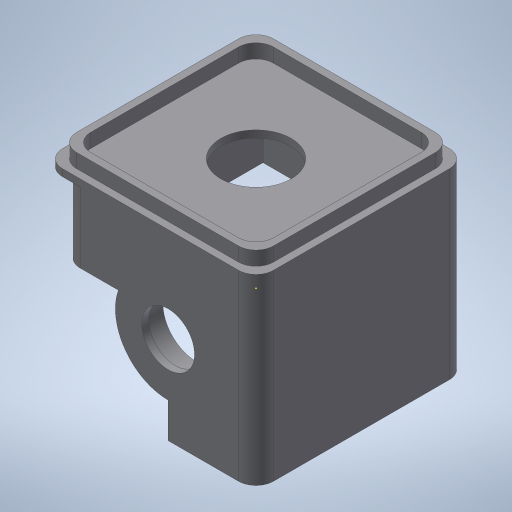
# Autodesk Inventor part: Pieza 2.3 final
Saved by Autodesk Inventor 2023.1 (Build 271208000, 208)
## iProperties
Created: 2022-10-20
Part Number: Pieza 2.3 final
Material: Generic
Document SubType Name: Modeling
Designer: User
Density: 1 g/cm^3
Appearance: Default
Author: User
Autodesk Inventor part; units mm, degrees
ref_plane "YZ Plane" through (0, 0, 0) normal (1, 0, 0) x (0, 1, 0)
ref_plane "XZ Plane" through (0, 0, 0) normal (0, 1, 0) x (-1, 0, 0)
ref_plane "XY Plane" through (0, 0, 0) normal (0, 0, 1) x (1, 0, 0)
sketch "Sketch1" plane through (0, 0, 0) normal (0, 1, 0) x (-1, 0, 0)
  line L0 (0, 0) -> (60, 0)
  line L1 (60, 0) -> (60, 60)
  line L2 (60, 60) -> (0, 60)
  line L3 (0, 60) -> (0, 0)
  dimension "d0" = 60
  dimension "d1" = 60
  constraints: 8 end point, 2 parallel, 1 horizontal, 1 perpendicular
  measures "d0" distance of L2.end L1.end
  measures "d1" distance of L1.end L0.end
extrude "Extrusion1" add sketch "Sketch1" along normal blind 2
sketch "Sketch2" plane through (0, 2, 0) normal (0, 1, 0) x (1, 0, 0)
  line L0 (-60, 0) -> (-60, -60) projected
  line L1 (-60, -60) -> (0, -60) projected
  line L2 (0, -60) -> (0, 0) projected
  line L3 (0, 0) -> (-60, 0) projected
  line L4 (-58, -2) -> (-58, -58)
  line L5 (-58, -58) -> (-2, -58)
  line L6 (-2, -58) -> (-2, -2)
  line L7 (-2, -2) -> (-58, -2)
  line L8 (-56, -4) -> (-56, -56)
  line L9 (-56, -56) -> (-4, -56)
  line L10 (-4, -56) -> (-4, -4)
  line L11 (-4, -4) -> (-56, -4)
  dimension "d4" = 2
  dimension "d5" = 2
  constraints: 16 end point, 6 other
  measures "d4" distance between parallel lines of L3 L7
  measures "d5" distance between parallel lines of L7 L11
extrude "Extrusion2" add sketch "Sketch2" along normal blind 4 contours L7 L6 L5 L4
sketch "Sketch3" plane through (0, 2, 0) normal (0, 1, 0) x (1, 0, 0)
  line L0 (0, 0) -> (-60, 0) construction
  line L1 (-60, 0) -> (-60, -60) construction
  line L2 (0, 0) -> (-60, -60) construction
  line L3 (-60, -60) -> (0, -60) construction
  line L4 (0, -60) -> (-60, 0) construction
  circle A0 centre (-30, -30) radius 10
  dimension "d8" = 20
  constraints: 4 end point, 1 centre point, 1 coincident, 1 midpoint
  measures "d8" diameter of A0
hole "Hole1" at (-30, 2, 30) direction (0, -1, 0) diameter 20 depth 8 tip angle 118
sketch "Sketch4" plane through (0, 0, 0) normal (0, -1, 0) x (1, 0, 0)
  circle A0 centre (-30, 30) radius 10 projected
  line L0 (-60, 0) -> (-60, 60) projected
  line L1 (0, 0) -> (-60, 0) projected
  line L2 (0, 60) -> (0, 0) projected
  line L3 (-60, 60) -> (0, 60) projected
  line L4 (0, 0) -> (-50, 0)
  line L5 (-50, 0) -> (-50, 8)
  line L6 (-50, 8) -> (0, 8)
  line L7 (0, 8) -> (0, 0)
  line L8 (0, 60) -> (-50, 60)
  line L9 (-50, 60) -> (-50, 52)
  line L10 (-50, 52) -> (0, 52)
  line L11 (0, 52) -> (0, 60)
  line L12 (0, 8) -> (-5, 8)
  line L13 (-5, 8) -> (-5, 52)
  line L14 (-5, 52) -> (0, 52)
  line L15 (0, 52) -> (0, 8)
  dimension "d16" = 50
  dimension "d17" = 8
  dimension "d18" = 50
  dimension "d19" = 8
  dimension "d20" = 5
  constraints: 24 end point, 6 parallel, 3 horizontal, 3 perpendicular, 1 point on line
  measures "d16" distance of L5.end L6.end
  measures "d17" distance of L4.end L5.end
  measures "d18" distance of L10.end L9.end
  measures "d19" distance of L9.end L8.end
  measures "d20" distance of L13.end L14.end
extrude "Extrusion3" add sketch "Sketch4" along normal blind 10 contours L5 L6 L2 L1 | L3 L2 L10 L9 | L6 L13 L10 L2
sketch "Sketch5" plane through (-5, 0, 52) normal (0, 0, -1) x (-1, 0, 0)
  line L0 (55, 0) -> (45, 0) projected
  line L1 (45, 0) -> (45, -10) projected
  line L2 (-5, -10) -> (45, -10) projected
  line L3 (-5, -10) -> (-5, 2) projected
  line L4 (55, 2) -> (-5, 2) projected
  line L5 (55, 0) -> (55, 2) projected
  line L6 (-5, -10) -> (45, -10) construction
  line L7 (-5, -10) -> (5, -10) construction
  line L8 (5, -10) -> (20, -10) construction
  line L9 (20, -10) -> (20, -25) construction
  circle A0 centre (20, -25) radius 15
  point P0 (-5, 0)
  dimension "d23" = 10
  dimension "d24" = 15
  dimension "d25" = 15
  dimension "d26" = 30
  constraints: 6 end point, 1 centre point, 1 coincident, 1 midpoint, 1 perpendicular, 1 point on line
  measures "d23" distance of L2.start L7.end
  measures "d24" distance of L7.end L8.end
  measures "d25" distance of L8.end L9.end
  measures "d26" diameter of A0
extrude "Extrusion4" add sketch "Sketch5" against normal blind 8 contours A0
sketch "Sketch6" plane through (-50, 0, 8) normal (0, 0, 1) x (1, 0, 0)
  line L0 (0, 0) -> (-10, 0) projected
  line L1 (-10, 0) -> (-10, 2) projected
  line L2 (50, 2) -> (-10, 2) projected
  line L3 (50, -10) -> (50, 2) projected
  line L4 (0, -10) -> (50, -10) projected
  line L5 (0, 0) -> (0, -10) projected
  line L6 (0, -10) -> (50, -10) construction
  line L7 (50, -10) -> (40, -10) construction
  line L8 (40, -10) -> (25, -10) construction
  line L9 (25, -10) -> (25, -25) construction
  circle A0 centre (25, -25) radius 15
  point P0 (50, 0)
  dimension "d29" = 10
  dimension "d30" = 15
  dimension "d31" = 15
  dimension "d32" = 30
  constraints: 6 end point, 1 centre point, 1 coincident, 1 midpoint, 1 perpendicular, 1 point on line
  measures "d29" distance of L3.start L7.end
  measures "d30" distance of L7.end L8.end
  measures "d31" distance of L8.end L9.end
  measures "d32" diameter of A0
extrude "Extrusion5" add sketch "Sketch6" against normal blind 8 contours A0
sketch "Sketch7" plane through (-25, -25, 52) normal (0, 0, -1) x (-1, 0, 0)
  circle A0 centre (0, 0) radius 15 projected
  circle A1 centre (0, 0) radius 13.5
  circle A2 centre (0, 0) radius 11.5
  circle A3 centre (0, 0) radius 15
  circle A4 centre (0, 0) radius 15 projected
  line L0 (0, -15) -> (0, 15)
  line L1 (15, 0) -> (-15, 0)
  line L2 (0, 0) -> (-12.9904, -7.5)
  line L3 (0, 0) -> (15, 0) construction
  line L4 (-12.9904, -7.5) -> (12.9904, 7.5)
  line L5 (0, 0) -> (-7.5, -12.9904)
  line L6 (0, 0) -> (15, 0) construction
  line L7 (-7.5, -12.9904) -> (7.5, 12.9904)
  line L8 (0, 0) -> (7.5, -12.9904)
  line L9 (0, 0) -> (15, 0) construction
  line L10 (7.5, -12.9904) -> (-7.5, 12.9904)
  line L11 (0, 0) -> (12.9904, -7.5)
  line L12 (0, 0) -> (15, 0) construction
  line L13 (12.9904, -7.5) -> (-12.9904, 7.5)
  point P0 (-25, 25)
  point P1 (11.6913, 6.75)
  point P2 (9.9593, 5.75)
  point P3 (11.5, 0)
  point P4 (13.5, 0)
  point P5 (5.75, 9.9593)
  point P6 (6.75, 11.6913)
  point P7 (0, 13.5)
  point P8 (0, 11.5)
  point P9 (-11.6913, 6.75)
  point P10 (-9.9593, 5.75)
  point P11 (-5.75, 9.9593)
  point P12 (-6.75, 11.6913)
  point P13 (-11.6913, -6.75)
  point P14 (-9.9593, -5.75)
  point P15 (-11.5, 0)
  point P16 (-13.5, 0)
  point P17 (-5.75, -9.9593)
  point P18 (-6.75, -11.6913)
  point P19 (0, -13.5)
  point P20 (0, -11.5)
  point P21 (11.6913, -6.75)
  point P22 (9.9593, -5.75)
  point P23 (5.75, -9.9593)
  point P24 (6.75, -11.6913)
  dimension "d35" = 1.5
  dimension "d36" = 2
  dimension "d37" = 30
  dimension "d38" = 150
  dimension "d39" = 120
  dimension "d40" = 60
  dimension "d41" = 30
  constraints: 28 end point, 5 horizontal, 4 equal length, 3 centre point, 3 point on line, 1 coincident, 1 vertical, 1 vertical alignment, 12 other
  measures "d36" radial gap between concentric circles of A1 A2
  measures "d37" diameter of A3
  measures "d38" angle of L2 L3
  measures "d39" angle of L5 L6
  measures "d40" angle of L8 L9
  measures "d41" angle of L11 L12
extrude "Extrusion6" cut sketch "Sketch7" against normal blind 5 contours L1 A2 L4 A1 | A1 L8 A2 L11 | L7 A2 L0 A1 | A1 L5 A2 L0 | A2 L2 A1 L1 | A2 L13 A1 L10
sketch "Sketch8" plane through (-25, -25, 8) normal (0, 0, 1) x (1, 0, 0)
  circle A0 centre (0, 0) radius 15
  circle A1 centre (0, 0) radius 13.5
  circle A2 centre (0, 0) radius 11.5
  circle A3 centre (0, 0) radius 15
  circle A4 centre (0, 0) radius 15
  line L0 (0, -15) -> (0, 15)
  line L1 (15, 0) -> (-15, 0)
  line L2 (0, 0) -> (-12.9904, -7.5)
  line L3 (0, 0) -> (15, 0) construction
  line L4 (-12.9904, -7.5) -> (12.9904, 7.5)
  line L5 (0, 0) -> (-7.5, -12.9904)
  line L6 (0, 0) -> (15, 0) construction
  line L7 (-7.5, -12.9904) -> (7.5, 12.9904)
  line L8 (0, 0) -> (7.5, -12.9904)
  line L9 (0, 0) -> (15, 0) construction
  line L10 (7.5, -12.9904) -> (-7.5, 12.9904)
  line L11 (0, 0) -> (12.9904, -7.5)
  line L12 (0, 0) -> (15, 0) construction
  line L13 (12.9904, -7.5) -> (-12.9904, 7.5)
  point P0 (25, 25)
  point P1 (-25, 25)
  point P2 (11.6913, 6.75)
  point P3 (9.9593, 5.75)
  point P4 (11.5, 0)
  point P5 (13.5, 0)
  point P6 (5.75, 9.9593)
  point P7 (6.75, 11.6913)
  point P8 (0, 13.5)
  point P9 (0, 11.5)
  point P10 (-11.6913, 6.75)
  point P11 (-9.9593, 5.75)
  point P12 (-5.75, 9.9593)
  point P13 (-6.75, 11.6913)
  point P14 (-11.6913, -6.75)
  point P15 (-9.9593, -5.75)
  point P16 (-11.5, 0)
  point P17 (-13.5, 0)
  point P18 (-5.75, -9.9593)
  point P19 (-6.75, -11.6913)
  point P20 (0, -13.5)
  point P21 (0, -11.5)
  point P22 (11.6913, -6.75)
  point P23 (9.9593, -5.75)
  point P24 (5.75, -9.9593)
  point P25 (6.75, -11.6913)
  point P26 (9.9593, -5.75)
  point P27 (11.6913, -6.75)
  point P28 (13.5, 0)
  point P29 (11.5, 0)
  point P30 (6.75, 11.6913)
  point P31 (5.75, 9.9593)
  point P32 (9.9593, 5.75)
  point P33 (11.6913, 6.75)
  point P34 (-6.75, 11.6913)
  point P35 (-5.75, 9.9593)
  point P36 (0, 11.5)
  point P37 (0, 13.5)
  point P38 (-9.9593, 5.75)
  point P39 (-11.6913, 6.75)
  point P40 (-13.5, 0)
  point P41 (-11.5, 0)
  point P42 (-6.75, -11.6913)
  point P43 (-5.75, -9.9593)
  point P44 (-9.9593, -5.75)
  point P45 (-11.6913, -6.75)
  point P46 (6.75, -11.6913)
  point P47 (5.75, -9.9593)
  point P48 (0, -11.5)
  point P49 (0, -13.5)
  dimension "d44" = 1.5
  dimension "d45" = 2
  dimension "d46" = 30
  dimension "d47" = 150
  dimension "d48" = 120
  dimension "d49" = 60
  dimension "d50" = 30
  constraints: 28 end point, 5 horizontal, 4 equal length, 3 centre point, 3 point on line, 1 coincident, 1 vertical, 1 vertical alignment, 14 other
  measures "d45" radial gap between concentric circles of A1 A2
  measures "d46" diameter of A3
  measures "d47" angle of L2 L3
  measures "d48" angle of L5 L6
  measures "d49" angle of L8 L9
  measures "d50" angle of L11 L12
extrude "Extrusion7" cut sketch "Sketch8" against normal blind 5 contours A1 L11 A2 L1 | L4 A2 L7 A1 | A1 L0 A2 L8 | L0 A2 L10 A1 | L1 A1 L13 A2 | A2 L5 A1 L2
sketch "Sketch9" plane through (-25, -25, 52) normal (0, 0, -1) x (-1, 0, 0)
  circle A0 centre (0, 0) radius 15 projected
  circle A1 centre (0, 0) radius 7.5
  point P0 (-25, 25)
  point P1 (0, 15)
  dimension "d53" = 15
  constraints: 1 centre point, 1 coincident, 1 vertical alignment
  measures "d53" diameter of A1
hole "Hole2" at (-25, -25, 52) direction (0, 0, 1) diameter 15 depth 8 tip angle 118
sketch "Sketch10" plane through (-25, -25, 8) normal (0, 0, 1) x (1, 0, 0)
  circle A0 centre (0, 0) radius 15 projected
  point P0 (25, 25)
  point P1 (0, 15)
  constraints: 1 coincident, 1 vertical alignment
hole "Hole3" at (-25, -25, 8) direction (0, 0, -1) diameter 15 depth 8 tip angle 118
sketch "Sketch11" plane through (-25, -25, 8) normal (0, 0, 1) x (1, 0, 0)
  circle A0 centre (0, 0) radius 7.5 projected
  circle A1 centre (0, 0) radius 15 projected
  circle A2 centre (0, 0) radius 9.5
  point P0 (25, 25)
  point P1 (0, 15)
  dimension "d68" = 2
  constraints: 1 centre point, 1 vertical alignment
  measures "d68" radial gap between concentric circles of A0 A2
extrude "Extrusion8" cut sketch "Sketch11" against normal blind 6 contours A2
sketch "Sketch12" plane through (-25, -25, 52) normal (0, 0, -1) x (-1, 0, 0)
  circle A0 centre (0, 0) radius 7.5 projected
  circle A1 centre (0, 0) radius 15 projected
  circle A2 centre (0, 0) radius 9.5
  point P0 (-25, 25)
  point P1 (0, 15)
  dimension "d71" = 2
  constraints: 1 centre point, 1 vertical alignment
  measures "d71" radial gap between concentric circles of A0 A2
extrude "Extrusion9" cut sketch "Sketch12" against normal blind 6 contours A2
sketch "Sketch13" plane through (-60, 2, 60) normal (0, 0, 1) x (1, 0, 0)
  point P0 (60, -2)
sketch "Sketch14" plane through (-60, 2, 60) normal (0, 0, 1) x (1, 0, 0)
  line L0 (0, -2) -> (10, -2) projected
  line L1 (10, -2) -> (10, -12) projected
  line L2 (35, -12) -> (10, -12) projected
  line L3 (60, -12) -> (35, -12) projected
  line L4 (60, -12) -> (60, 0) projected
  line L5 (0, 0) -> (60, 0) projected
  line L6 (0, -2) -> (0, 0) projected
  arc A0 (44.9593, -21.25) -> (40.75, -17.0407) centre (35, -27) ccw projected
  circle A1 centre (35, -27) radius 15 projected
  line L7 (60, -12) -> (60, 0) projected
  line L8 (60, -12) -> (35, -12)
  line L9 (35, -42) -> (35, -52)
  line L10 (35, -52) -> (60, -52)
  line L11 (60, -52) -> (60, -12)
  arc A2 (35, -42) -> (35, -12) centre (35, -27) ccw
  point P0 (60, -2)
  dimension "d74" = 25
  dimension "d75" = 40
  constraints: 8 end point, 2 parallel, 2 point on circle, 1 centre point, 1 coincident, 1 horizontal, 1 perpendicular, 1 other
  measures "d74" distance of L10.end L9.end
  measures "d75" distance of L9.end L8.end
extrude "Extrusion10" add sketch "Sketch14" against normal blind 8 contours L3 L11 L10 L9 A1
sketch "Sketch15" plane through (0, 2, 0) normal (0, 0, -1) x (-1, 0, 0)
  line L0 (50, -2) -> (60, -2) projected
  line L1 (60, -2) -> (60, 0) projected
  line L2 (0, 0) -> (60, 0) projected
  line L3 (0, -12) -> (0, 0) projected
  line L4 (25, -12) -> (0, -12) projected
  line L5 (50, -12) -> (25, -12) projected
  line L6 (50, -2) -> (50, -12) projected
  circle A0 centre (25, -27) radius 15 projected
  line L7 (0, -52) -> (25, -52) projected
  line L8 (25, -12) -> (0, -12)
  line L9 (0, -12) -> (0, -52)
  line L10 (0, -52) -> (25, -52)
  circle A1 centre (25, -27) radius 7.5 projected
  arc A2 (25, -12) -> (25, -42) centre (25, -27) ccw
  line L11 (25, -52) -> (25, -42)
  point P0 (0, -2)
  constraints: 8 end point, 2 parallel, 2 point on circle, 1 centre point, 1 coincident, 1 horizontal, 1 perpendicular, 2 other
extrude "Extrusion11" add sketch "Sketch15" against normal blind 8 contours A0 L11 L7 L9 L4
sketch "Sketch16" plane through (0, -10, 0) normal (0, -1, 0) x (1, 0, 0)
  line L0 (-4, 56) -> (-4, 4) projected
  line L1 (0, 8) -> (0, 52) projected
  line L2 (-5, 52) -> (-5, 8) projected
  line L3 (-25, 8) -> (0, 8) projected
  line L4 (0, 52) -> (-25, 52) projected
  line L5 (-5, 8) -> (-5, 52) projected
  line L6 (0, 8) -> (-5, 8)
  line L7 (-5, 8) -> (-5, 52)
  line L8 (-5, 52) -> (0, 52)
  line L9 (0, 52) -> (0, 8)
  point P0 (0, 0)
  constraints: 8 end point, 2 parallel, 1 horizontal, 1 perpendicular
extrude "Extrusion12" add sketch "Sketch16" along normal blind 40
sketch "Sketch17" plane through (0, 0, 0) normal (0, -1, 0) x (1, 0, 0)
  line L0 (-50, 52) -> (-50, 60) projected
  line L1 (-60, 60) -> (-50, 60) projected
  line L2 (-60, 0) -> (-60, 60) projected
  line L3 (-50, 0) -> (-60, 0) projected
  line L4 (-50, 0) -> (-50, 8) projected
  line L5 (-50, 8) -> (-5, 8) projected
  line L6 (-5, 8) -> (-5, 52) projected
  line L7 (-5, 52) -> (-50, 52) projected
  circle A0 centre (-30, 30) radius 10 projected
  line L8 (-50, 60) -> (-50, 52) projected
  line L9 (-50, 60) -> (-55, 60)
  line L10 (-55, 60) -> (-55, 0)
  line L11 (-55, 0) -> (-50, 0)
  line L12 (-50, 0) -> (-50, 60)
  point P0 (0, 0)
  dimension "d82" = 5
  dimension "d83" = 60
  constraints: 8 end point, 2 parallel, 1 horizontal, 1 perpendicular
  measures "d82" distance of L11.end L10.end
  measures "d83" distance of L10.end L9.end
extrude "Extrusion13" add sketch "Sketch17" along normal blind 20 contours L12 L4 L3 L10 L1 L0
sketch "Sketch18" plane through (0, 2, 0) normal (0, 0, -1) x (-1, 0, 0)
  circle A0 centre (25, -27) radius 7.5 projected
  line L0 (55, -2) -> (60, -2) projected
  line L1 (60, -2) -> (60, 0) projected
  line L2 (0, 0) -> (60, 0) projected
  line L3 (0, -52) -> (0, 0) projected
  line L4 (0, -52) -> (25, -52) projected
  line L5 (25, -52) -> (25, -42) projected
  arc A1 (25, -42) -> (25, -12) centre (25, -27) ccw projected
  line L6 (50, -12) -> (25, -12) projected
  line L7 (50, -12) -> (50, -22) projected
  line L8 (55, -22) -> (50, -22) projected
  line L9 (55, -2) -> (55, -22) projected
  line L10 (50, -12) -> (50, -22) projected
  line L11 (50, -12) -> (25, -12)
  line L12 (50, -22) -> (50, -12)
  arc A2 (39.1421, -22) -> (25, -12) centre (25, -27) ccw
  line L13 (39.1421, -22) -> (50, -22)
  point P0 (0, -2)
  constraints: 7 end point, 2 point on circle, 1 centre point, 1 coincident, 1 horizontal, 1 parallel
extrude "Extrusion14" add sketch "Sketch18" against normal blind 8 contours L13 A1 L6 L7
sketch "Sketch19" plane through (-60, 2, 60) normal (0, 0, 1) x (1, 0, 0)
  circle A0 centre (35, -27) radius 7.5 projected
  arc A1 (35, -12) -> (35, -42) centre (35, -27) ccw projected
  line L0 (35, -42) -> (35, -52) projected
  line L1 (35, -52) -> (60, -52) projected
  line L2 (60, -52) -> (60, 0) projected
  line L3 (0, 0) -> (60, 0) projected
  line L4 (0, -2) -> (0, 0) projected
  line L5 (0, -2) -> (5, -2) projected
  line L6 (5, -2) -> (5, -22) projected
  line L7 (10, -22) -> (5, -22) projected
  line L8 (10, -12) -> (10, -22) projected
  line L9 (35, -12) -> (10, -12) projected
  line L10 (35, -22) -> (35, -19.5)
  line L11 (35, -12) -> (10, -12)
  line L12 (10, -12) -> (10, -22)
  arc A2 (35, -12) -> (20.8579, -22) centre (35, -27) ccw
  line L13 (10, -22) -> (20.8579, -22)
  point P0 (60, -2)
  constraints: 9 end point, 2 parallel, 2 point on circle, 1 centre point, 1 coincident, 1 horizontal, 1 perpendicular, 1 vertical alignment, 1 other
extrude "Extrusion15" add sketch "Sketch19" against normal blind 8 contours A1 L13 L8 L9
fillet "Fillet1" radius 5 14 edges at (0, -24, 0) (-55, -10, 0) (-55, -10, 60) (0, -24, 60) (-2, 4, 58) (-2, 4, 2) (-60, 1, 0) (-58, 4, 2) (-60, 1, 60) (-58, 4, 58) (-56, 4, 56) (-56, 4, 4) (-4, 4, 56) (-4, 4, 4)
body "Solid1"
